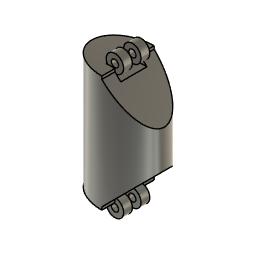
thumb1 v1 (Autodesk Fusion 360 design; units mm, degrees)
Autodesk Fusion 360 part; units mm, degrees
sketch "Sketch1" plane through (0, 0, 0) normal (0, 0, 1) x (1, 0, 0)
  ellipse E0 centre (0, 0) end of major axis (12.5, 0) minor radius 9
  line L0 (-12.5, 0) -> (12.5, 0) construction
  line L1 (0, -9) -> (0, 9) construction
  dimension "d1" = 25
  dimension "d2" = 18
  constraint coincident E0 L0.start
  constraint coincident E0 L0.end
  constraint coincident E0 L1.start
  constraint coincident E0 L1.end
  constraint coincident E0.centre origin
  constraint horizontal L0
  measures "d1" distance of E0
extrude "Extrude1" add sketch "Sketch1" along normal blind 40
sketch "Sketch2" plane through (0, 0, 0) normal (0, 1, 0) x (1, 0, 0)
  line L0 (-12.5, 0) -> (12.5, 0)
  line L1 (0, 0) -> (0, -1)
  line L2 (0, -1) -> (15, -16)
  line L3 (15, -16) -> (15, 0)
  line L4 (15, 0) -> (0, 0)
  line L5 (-12.5, -40) -> (12.5, -40)
  line L6 (0, -40) -> (0, -39)
  line L7 (0, -39) -> (15.8611, -23.1389)
  line L8 (0, -39) -> (22.431, -39) construction
  line L9 (15.8611, -23.1389) -> (15.8611, -40)
  line L10 (15.8611, -40) -> (0, -40)
  dimension "d5" = 1
  dimension "d6" = 1
  dimension "d7" = 45
  constraint coincident L1.start L4.end
  constraint perpendicular L0 L1
  constraint vertical L3
  constraint perpendicular L1 L4
  constraint midpoint L5 L6.start
  constraint perpendicular L5 L6
  constraint horizontal L8
  constraint perpendicular L8 L9
  constraint perpendicular L6 L10
  measures "d5" distance of L1.start L1.end
  measures "d6" distance of L6.start L6.end
  measures "d7" angle of L7 L8
extrude "Extrude2" cut sketch "Sketch2" along normal mid plane 200
sketch "Sketch3" plane through (0, 0, 0) normal (1, 0, 0) x (0, 1, 0)
  line L0 (-9, 40) -> (-9, 39)
  line L1 (-9, 39) -> (9, 39)
  line L2 (9, 39) -> (9, 40)
  line L3 (9, 40) -> (-9, 40)
  line L4 (0, 0) -> (4.5, 0)
  line L5 (4.5, 0) -> (4.5, 3)
  line L6 (4.5, 3) -> (0, 3)
  line L7 (0, 3) -> (0, 0)
  line L8 (0, 0) -> (-4.5, 0)
  line L9 (-4.5, 0) -> (-4.5, 3)
  line L10 (-4.5, 3) -> (0, 3)
  line L11 (0, 3) -> (0, 0)
  line L12 (0, 40) -> (4.5, 40)
  line L13 (4.5, 40) -> (4.5, 37)
  line L14 (4.5, 37) -> (0, 37)
  line L15 (0, 37) -> (0, 40)
  line L16 (0, 40) -> (-4.5, 40)
  line L17 (-4.5, 40) -> (-4.5, 37)
  line L18 (-4.5, 37) -> (0, 37)
  line L19 (0, 37) -> (0, 40)
  dimension "d10" = 4.5
  dimension "d11" = 3
  dimension "d12" = 4.5
  dimension "d13" = 3
  dimension "d14" = 4.5
  dimension "d15" = 3
  dimension "d16" = 3
  constraint horizontal L4
  constraint vertical L5
  constraint horizontal L6
  constraint vertical L7
  constraint coincident L4.start L7.end
  constraint horizontal L8
  constraint vertical L9
  constraint horizontal L10
  constraint vertical L11
  constraint horizontal L12
  constraint vertical L13
  constraint horizontal L14
  constraint vertical L15
  constraint midpoint L3 L12.start
  constraint horizontal L16
  constraint vertical L17
  constraint horizontal L18
  constraint vertical L19
  measures "d10" distance of L4.start L4.end
  measures "d11" distance of L4.start L6.end
  measures "d12" distance of L4.start L8.end
  measures "d13" distance of L4.start L6.end
  measures "d14" distance of L12.start L12.end
  measures "d15" distance of L12.start L14.end
  measures "d16" distance of L12.start L14.end
extrude "Extrude3" cut sketch "Sketch3" along normal mid plane 6 contours L1 L3 L15 L16 L17 L19 | L1 L15 L17 L18 L19 | L1 L3 L12 L13 L15 L19 | L1 L13 L14 L15 L19 | L4 L5 L6 L7 L11 | L7 L8 L9 L10 L11
ref_plane "WorkPlane1" through (-0.5, 0, 1.5) normal (0, 1, 0) x (0, 0, 1)
sketch "Sketch4" plane through (0, 0, 0) normal (0, 1, 0) x (1, 0, 0)
  line L0 (-12.5, 0) -> (0, 0)
  circle A0 centre (0, 1.5) radius 1.25
  circle A1 centre (0, 1.5) radius 3
  circle A2 centre (0, -41.5) radius 1.25
  circle A3 centre (0, -41.5) radius 3
  point P0 (0, -40)
  dimension "d19" = 2.5
  dimension "d20" = 6
  dimension "d21" = 1.5
  dimension "d22" = 2.5
  dimension "d23" = 6
  dimension "d24" = 1.5
  constraint concentric A0 A1
  constraint concentric A2 A3
  measures "d19" diameter of A0
  measures "d20" diameter of A1
  measures "d21" distance of L0.end A0.centre
  measures "d22" diameter of A2
  measures "d23" diameter of A3
  measures "d24" distance of A2.centre P0
extrude "Extrude4" add sketch "Sketch4" along normal mid plane 9
extrude "Extrude5" cut sketch "Sketch4" along normal mid plane 3
move_body "Move1" bodies 1 to x (1, 0, 0) y (0, 1, 0) z (0, 0, 1) at (0, 180, 0)
